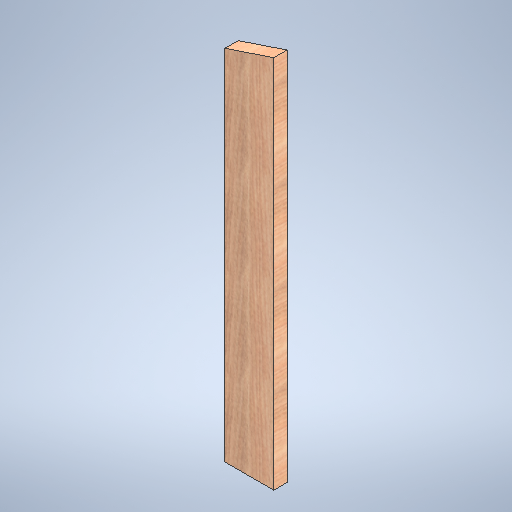
# Autodesk Inventor part: Stud_With_Height_42.5_Inches
Saved by Autodesk Inventor 2025 (Build 290162010, 162A)
## iProperties
Created: 2024-09-16
Part Number: Stud_With_Height_42.5_Inches
Material: Wood (Birch)
Document SubType Name: Modeling
Designer: Tom
Density: 0.55 g/cm^3
Appearance: Birch - Natural Polished
Author: Tom
Autodesk Inventor part; units mm, degrees
ref_plane "YZ Plane" through (0, 0, 0) normal (1, 0, 0) x (0, 1, 0)
ref_plane "XZ Plane" through (0, 0, 0) normal (0, 1, 0) x (-1, 0, 0)
ref_plane "XY Plane" through (0, 0, 0) normal (0, 0, 1) x (1, 0, 0)
sketch "Sketch1" plane through (0, 0, 0) normal (0, 0, 1) x (1, 0, 0)
  line L0 (0, 0) -> (139.7, 0)
  line L1 (139.7, 0) -> (139.7, 1071.5625)
  line L2 (0, 1024.9728) -> (0, 0)
  line L3 (139.7, 1071.5625) -> (0, 1024.9728)
  line L4 (139.7, 1071.5625) -> (-3073.4, 1071.5625)
  line L5 (-3073.4, 1071.5625) -> (-3073.4, 0)
  line L6 (-3073.4, 0) -> (139.7, 1071.5625)
  dimension "d3" = 139.7
  dimension "d6" = 1071.5625
  dimension "d9" = 3213.1
  dimension "d10" = 1071.5625
  constraints: 14 end point, 2 horizontal, 2 perpendicular, 1 collinear, 1 parallel
  measures "d3" distance of L0.start L0.end
  measures "d6" distance of L0.end L1.end
  measures "d9" distance of L1.end L4.end
  measures "d10" distance of L4.end L5.end
extrude "Extrusion1" add sketch "Sketch1" along normal blind 38.1 contours L2 L3 L1 L0
body "Solid1"
